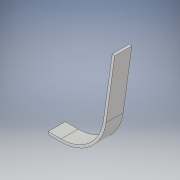
# Autodesk Inventor part: ball-reload-left
Saved by Autodesk Inventor 2017 (Build 210142000, 142)
## iProperties
Created: 2017-03-05
Part Number: ball-reload-left
Material: Generic
Document SubType Name: Modeling
Designer: John
Density: 1 g/cm^3
Appearance: Default
Author: John
Autodesk Inventor part; units mm, degrees
note: some values were not read from the file. Chosen so that the rebuilt part matches the saved one: bend side of "Bend Part1".
ref_plane "YZ Plane" through (0, 0, 0) normal (1, 0, 0) x (0, 1, 0)
ref_plane "XZ Plane" through (0, 0, 0) normal (0, 1, 0) x (-1, 0, 0)
ref_plane "XY Plane" through (0, 0, 0) normal (0, 0, 1) x (1, 0, 0)
sketch "Sketch2" plane through (0, 0, 0) normal (0, 1, 0) x (-1, 0, 0)
  line L0 (0, 0) -> (-160, 0)
  line L1 (-160, 0) -> (-160, -20)
  line L2 (-160, -20) -> (0, -20)
  line L3 (0, -20) -> (0, 0)
  dimension "d0" = 160
  dimension "d1" = 20
  constraints: 8 end point, 2 parallel, 1 horizontal, 1 perpendicular
  measures "d0" distance of L2.end L1.end
  measures "d1" distance of L1.end L0.end
extrude "Extrusion1" add sketch "Sketch2" along normal blind 3
sketch "Sketch3" plane through (0, 3, 0) normal (0, 1, 0) x (1, 0, 0)
  line L0 (160, 20) -> (0, 20) projected
  line L1 (160, 0) -> (160, 20) projected
  line L2 (160, 20) -> (160, 0)
  line L3 (15, 20) -> (15, 0)
  line L4 (0, 0) -> (160, 0) projected
  line L5 (0, 20) -> (0, 0) projected
  dimension "d8" = 15
  constraints: 4 end point, 2 point on line, 2 vertical
  measures "d8" distance between parallel lines of L5 L3
bend part "Bend Part1" radius 50 angle 82 line through (15, 3, -20) along (0, 0, 1) centre toward (0, 1, 0) moving side (1, 0, 0) both sides no
body "Solid1"
